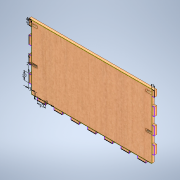
# Autodesk Inventor part: DoosjeVoorkant
Saved by Autodesk Inventor 2021 (Build 250183000, 183)
## iProperties
Created: 2021-03-11
Part Number: DoosjeVoorkant
Material: Wood (Cherry)
Document SubType Name: Modeling
Designer: ZiweZhang
Density: 0.63 g/cm^3
Appearance: Cherry - Natural Low Gloss
Author: ZiweZhang
Autodesk Inventor part; units mm, degrees
ref_plane "YZ Plane" through (0, 0, 0) normal (1, 0, 0) x (0, 1, 0)
ref_plane "XZ Plane" through (0, 0, 0) normal (0, 1, 0) x (-1, 0, 0)
ref_plane "XY Plane" through (0, 0, 0) normal (0, 0, 1) x (1, 0, 0)
sketch "Sketch1" plane through (0, 0, 0) normal (0, 0, 1) x (1, 0, 0)
  line L0 (0, 0) -> (144, 0)
  line L1 (144, 0) -> (144, 77)
  line L2 (144, 77) -> (0, 77)
  line L3 (0, 77) -> (0, 0)
  dimension "d0" = 144
  dimension "d1" = 77
  constraints: 8 end point, 2 parallel, 1 horizontal, 1 perpendicular
  measures "d0" distance of L2.end L1.end
  measures "d1" distance of L1.end L0.end
extrude "Extrusion1" add sketch "Sketch1" along normal blind 3
sketch "Sketch2" plane through (0, 0, 3) normal (0, 0, 1) x (1, 0, 0)
  line L0 (144, 77) -> (0, 77) projected
  line L1 (0, 0) -> (144, 0) projected
  line L2 (0, 77) -> (144, 77)
  line L3 (144, 77) -> (144, 0)
  line L4 (144, 0) -> (0, 0)
  line L5 (0, 0) -> (0, 77)
  line L6 (7, 0) -> (7, -3)
  line L7 (7, -3) -> (17, -3)
  line L8 (17, -3) -> (17, 0)
  line L9 (27, 0) -> (27, -3)
  line L10 (27, -3) -> (37, -3)
  line L11 (37, -3) -> (37, 0)
  line L12 (47, 0) -> (47, -3)
  line L13 (47, -3) -> (57, -3)
  line L14 (57, -3) -> (57, 0)
  line L15 (67, 0) -> (67, -3)
  line L16 (67, -3) -> (77, -3)
  line L17 (77, -3) -> (77, 0)
  line L18 (87, 0) -> (87, -3)
  line L19 (87, -3) -> (97, -3)
  line L20 (97, -3) -> (97, 0)
  line L21 (107, 0) -> (107, -3)
  line L22 (107, -3) -> (117, -3)
  line L23 (117, -3) -> (117, 0)
  line L24 (127, 0) -> (127, -3)
  line L25 (127, -3) -> (137, -3)
  line L26 (137, -3) -> (137, 0)
  line L27 (0, 77) -> (0, 0) projected
  line L28 (0, 10) -> (-3, 10)
  line L29 (-3, 10) -> (-3, 20)
  line L30 (-3, 20) -> (0, 20)
  line L31 (-3, 40) -> (0, 40)
  line L32 (-3, 30) -> (-3, 40)
  line L33 (0, 30) -> (-3, 30)
  line L34 (-3, 60) -> (0, 60)
  line L35 (-3, 50) -> (-3, 60)
  line L36 (0, 50) -> (-3, 50)
  line L37 (144, 77) -> (0, 77) projected
  line L38 (0, 77) -> (-3, 77)
  line L39 (-3, 77) -> (-3, 70)
  line L40 (-3, 70) -> (0, 70)
  line L41 (144, 0) -> (144, 77) projected
  line L42 (144, 77) -> (147, 77)
  line L43 (147, 77) -> (147, 70)
  line L44 (147, 70) -> (144, 70)
  line L45 (144, 0) -> (144, 77) projected
  line L46 (144, 60) -> (147, 60)
  line L47 (147, 60) -> (147, 50)
  line L48 (147, 50) -> (144, 50)
  line L49 (144, 40) -> (147, 40)
  line L50 (147, 40) -> (147, 30)
  line L51 (147, 30) -> (144, 30)
  line L52 (144, 20) -> (147, 20)
  line L53 (147, 20) -> (147, 10)
  line L54 (147, 10) -> (144, 10)
  dimension "d4" = 3
  dimension "d5" = 10
  dimension "d8" = 20
  dimension "d13" = 3
  dimension "d14" = 10
  dimension "d17" = 20
  dimension "d22" = 3
  dimension "d23" = 7
  dimension "d24" = 3
  constraints: 98 end point, 18 point on line, 16 perpendicular, 3 horizontal, 3 parallel, 1 vertical, 56 other
  measures "d4" distance of L6.start L6.end
  measures "d5" distance of L6.end L7.end
  measures "d8" distance of L6.start L9.start
  measures "d13" distance of L28.start L28.end
  measures "d14" distance of L28.end L29.end
  measures "d17" distance of L29.end L31.start
  measures "d22" distance of L0.end L38.end
  measures "d23" distance of L38.end L39.end
  measures "d24" distance of L0.start L42.end
extrude "Extrusion2" add sketch "Sketch2" against normal blind 3 contours L42 L43 L44 L3 | L5 L40 L39 L38 | L46 L47 L48 L3 | L5 L36 L35 L34 | L49 L50 L51 L3 | L5 L33 L32 L31 | L52 L53 L54 L3 | L5 L28 L29 L30 | L26 L25 L24 L1 | L1 L8 L7 L6 | L23 L22 L21 L1 | L1 L11 L10 L9 | L20 L19 L18 L1 | L1 L14 L13 L12 | L17 L16 L15 L1
sketch "Sketch3" plane through (0, 0, 3) normal (0, 0, 1) x (1, 0, 0)
  line L0 (0, 74) -> (7, 74)
  line L1 (7, 74) -> (7, 71)
  line L2 (7, 71) -> (0, 71)
  line L3 (0, 71) -> (0, 74)
  line L4 (137, 74) -> (144, 74)
  line L5 (144, 74) -> (144, 71)
  line L6 (144, 71) -> (137, 71)
  line L7 (137, 71) -> (137, 74)
  line L8 (0, 33) -> (7, 33)
  line L9 (7, 33) -> (7, 30)
  line L10 (7, 30) -> (0, 30)
  line L11 (0, 30) -> (0, 33)
  line L12 (137, 33) -> (144, 33)
  line L13 (144, 33) -> (144, 30)
  line L14 (144, 30) -> (137, 30)
  line L15 (137, 30) -> (137, 33)
  point P0 (0, 0)
  dimension "d27" = 7
  dimension "d28" = 3
  dimension "d31" = 137
  dimension "d34" = 41
  constraints: 32 end point, 3 perpendicular, 2 collinear, 2 horizontal, 1 vertical, 22 other
  measures "d27" distance of L0.start L0.end
  measures "d28" distance of L0.end L1.end
  measures "d31" distance of L0.start L4.start
  measures "d34" distance of L0.start L8.start
extrude "Extrusion3" cut sketch "Sketch3" against normal through all
body "Solid1"
